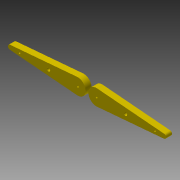
# Autodesk Inventor part: Eyebrows
Saved by Autodesk Inventor 2015 (Build 190159000, 159)
## iProperties
Created: 2015-03-18
Part Number: Eyebrows
Material: Generic
Document SubType Name: Modeling
Designer: ChristopherEvan
Density: 1 g/cm^3
Appearance: Default
Author: ChristopherEvan
Autodesk Inventor part; units mm, degrees
note: some values were not read from the file. Chosen so that the rebuilt part matches the saved one: sketch regions of "Extrusion1".
ref_plane "YZ Plane" through (0, 0, 0) normal (1, 0, 0) x (0, 1, 0)
ref_plane "XZ Plane" through (0, 0, 0) normal (0, 1, 0) x (-1, 0, 0)
ref_plane "XY Plane" through (0, 0, 0) normal (0, 0, 1) x (1, 0, 0)
sketch "Sketch1" plane through (0, 0, 0) normal (0, 0, 1) x (1, 0, 0)
  circle A0 centre (-30.6, 0) radius 0.5
  circle A1 centre (-1.4, 0) radius 0.5
  circle A2 centre (22.5792, 0) radius 0.85
  circle A3 centre (7.9792, 0) radius 0.5
  circle A4 centre (37.1792, 0) radius 0.5
  circle A5 centre (-1.4, 0) radius 4
  circle A6 centre (7.9792, 0) radius 4
  circle A7 centre (-35.2, 0) radius 1.1
  circle A8 centre (41.7792, 0) radius 1.1
  line L0 (-1.4, 4) -> (-35.2939, 1.096)
  line L1 (-1.4, -4) -> (-35.2939, -1.096)
  line L2 (7.9792, 4) -> (41.8731, 1.096)
  line L3 (7.9792, -4) -> (41.8731, -1.096)
  circle A9 centre (-16, 0) radius 0.85
  dimension "d0" = 8
  dimension "d1" = 8
  constraints: 10 centre point, 8 end point, 8 point on circle, 4 tangent, 2 coincident
  measures "d0" diameter of A5
  measures "d1" diameter of A6
extrude "Extrusion1" add sketch "Sketch1" along normal blind 3 contours A5 L1 L0 | A5 L1 A7 L0 | A7 | L2 A6 L3 | A6 L2 | L3 A6 | L2 A8 L3 A6 | A8
body "Solid1"
